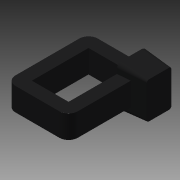
# Autodesk Inventor part: fastener_04
Saved by Autodesk Inventor 2013 (Build 170138000, 138)
## iProperties
Shininess: 41.0
Created: 2014-04-23
Part Number: fastener_04
Document SubType Name: Modeling
Designer: Noa Izumi
Material: Default
Density: 1 g/cm^3
Density: 0.0
Volumn: 0.0
Area: 0.0
PropertySet Name: Model Information
Control State: 0
Master: False
Checked Out: False
Author: Noa Izumi
Autodesk Inventor part; units mm, degrees
ref_plane "YZ Plane" through (0, 0, 0) normal (1, 0, 0) x (0, 1, 0)
ref_plane "XZ Plane" through (0, 0, 0) normal (0, 1, 0) x (-1, 0, 0)
ref_plane "XY Plane" through (0, 0, 0) normal (0, 0, 1) x (1, 0, 0)
sketch "Sketch1" plane through (0, 0, 0) normal (0, 0, 1) x (1, 0, 0)
  line L0 (0, 0) -> (4, 0)
  line L1 (4, 0) -> (4, 6.175)
  line L2 (4, 6.175) -> (0, 6.175)
  line L3 (0, 6.175) -> (0, 0)
  line L4 (-0.4, -1.4) -> (4.4, -1.4)
  line L5 (5.4, -0.4) -> (5.4, 7.575)
  line L6 (5.4, 7.575) -> (-0.4, 7.575)
  line L7 (-1.4, 6.575) -> (-1.4, -0.4)
  arc A0 (-0.4, 7.575) -> (-1.4, 6.575) centre (-0.4, 6.575) ccw
  arc A1 (-1.4, -0.4) -> (-0.4, -1.4) centre (-0.4, -0.4) ccw
  arc A2 (4.4, -1.4) -> (5.4, -0.4) centre (4.4, -0.4) ccw
  point P0 (-1.4, -1.4)
  point P1 (5.4, -1.4)
  point P2 (-1.4, 7.575)
  dimension "d0" = 4
  dimension "d1" = 6.175
  dimension "d2" = 1.4
  dimension "d5" = 1
  constraints: 16 end point, 6 point on circle, 6 point on line, 6 tangent, 4 parallel, 3 centre point, 2 equal radius, 2 perpendicular, 1 horizontal, 3 other
  measures "d0" distance of L0.start L0.end
  measures "d1" distance of L0.end L1.end
  measures "d2" distance between parallel lines of L3 L7
  measures "d5" radius of A0
extrude "Extrusion1" add sketch "Sketch1" along normal blind 2.5
sketch "草圖3" plane through (4, 6.175, 0) normal (-1, 0, 0) x (0, 0, 1)
  line L0 (0, -6.175) -> (0, 0) projected
  line L1 (-0.5, 2.3) -> (3, 2.3)
  line L2 (3.5, 1.8) -> (3.5, -0.4)
  line L3 (3, -0.9) -> (-0.5, -0.9)
  line L4 (-1, -0.4) -> (-1, 1.8)
  line L5 (0, -7.575) -> (2.5, -7.575) projected
  arc A0 (-0.5, 2.3) -> (-1, 1.8) centre (-0.5, 1.8) ccw
  arc A1 (-1, -0.4) -> (-0.5, -0.9) centre (-0.5, -0.4) ccw
  arc A2 (3, -0.9) -> (3.5, -0.4) centre (3, -0.4) ccw
  arc A3 (3.5, 1.8) -> (3, 2.3) centre (3, 1.8) ccw
  point P0 (-1, 2.3)
  point P1 (3.5, -0.9)
  point P2 (3.5, 2.3)
  dimension "d13" = 4.5
  dimension "d15" = 3.2
  dimension "d16" = 1
  dimension "d17" = 6.675
  dimension "d18" = 0.5
  constraints: 8 end point, 8 point on circle, 8 tangent, 6 point on line, 4 centre point, 3 equal radius, 2 parallel, 1 horizontal, 1 perpendicular
  measures "d13" distance of point (-1, 2.3) point (3.5, 2.3)
  measures "d15" distance of point (3.5, 2.3) point (3.5, -0.9)
  measures "d16" distance between parallel lines of L0 L4
  measures "d17" distance between parallel lines of L5 L3
  measures "d18" radius of A0
extrude "擠出3" add sketch "草圖3" against normal blind 3 draft -5
